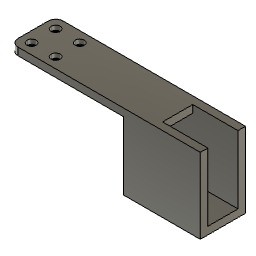
_Motor mount.45995b92-4b40-4a62-bec2-e495f78e715f (Autodesk Fusion 360 design; units mm, degrees)
Autodesk Fusion 360 part; units mm, degrees
sketch "Sketch1" plane through (0, 0, 0) normal (0, 0, 1) x (1, 0, 0)
  line L0 (0, 0) -> (51, 0)
  line L1 (51, 0) -> (51, -30)
  line L2 (51, -30) -> (0, -30)
  line L3 (0, -30) -> (0, 0)
  dimension "d1" = 51
  dimension "d2" = 30
  constraint horizontal L0
  constraint vertical L1
  constraint horizontal L2
  constraint vertical L3
  constraint coincident L0.start L3.end
  measures "d1" distance of L0.start L0.end
  measures "d2" distance of L0.start L2.end
extrude "Extrude1" add sketch "Sketch1" along normal blind 50
sketch "Sketch2" plane through (51, 0, 0) normal (1, 0, 0) x (0, 1, 0)
  line L0 (-30, 0) -> (0, 0)
  line L1 (0, 0) -> (0, 50)
  line L2 (0, 50) -> (-30, 50)
  line L3 (-30, 50) -> (-30, 0)
  line L4 (-5, 5) -> (-25, 5)
  line L5 (-25, 5) -> (-25, 45)
  line L6 (-25, 45) -> (-5, 45)
  line L7 (-5, 45) -> (-5, 5)
  dimension "d5" = 20
  dimension "d6" = 40
  constraint horizontal L4
  constraint vertical L5
  constraint horizontal L6
  constraint vertical L7
  measures "d5" distance of L4.start L4.end
  measures "d6" distance of L4.start L6.end
extrude "Extrude2" cut sketch "Sketch2" against normal blind 46 contours L4 L5 L6 L7
sketch "Sketch3" plane through (0, 0, 50) normal (0, 0, 1) x (-1, 0, 0)
  line L0 (0, 30) -> (-51, 30)
  line L1 (-51, 30) -> (-51, 0)
  line L2 (-51, 0) -> (0, 0)
  line L3 (0, 0) -> (0, 30)
  line L4 (-51, 5) -> (-21, 5)
  line L5 (-21, 5) -> (-21, 25)
  line L6 (-21, 25) -> (-51, 25)
  line L7 (-51, 25) -> (-51, 5)
  dimension "d9" = 30
  dimension "d10" = 20
  constraint horizontal L4
  constraint vertical L5
  constraint horizontal L6
  constraint vertical L7
  constraint coincident L1 L4.start
  measures "d9" distance of L4.start L4.end
  measures "d10" distance of L4.start L6.end
extrude "Extrude3" cut sketch "Sketch3" against normal blind 6 contours L1 L4 L5 L6 L7
sketch "Sketch4" plane through (0, 0, 50) normal (0, 0, 1) x (-1, 0, 0)
  line L0 (-51, 25) -> (-21, 25)
  line L1 (-21, 25) -> (-21, 5)
  line L2 (-21, 5) -> (-51, 5)
  line L3 (-51, 5) -> (-51, 0)
  line L4 (-51, 0) -> (0, 0)
  line L5 (0, 0) -> (0, 30)
  line L6 (0, 30) -> (-51, 30)
  line L7 (-51, 30) -> (-51, 25)
  line L8 (0, 0) -> (75, 0)
  line L9 (75, 0) -> (75, 30)
  line L10 (75, 30) -> (0, 30)
  line L11 (0, 30) -> (0, 0)
  dimension "d13" = 75
  dimension "d14" = 30
  constraint horizontal L8
  constraint vertical L9
  constraint horizontal L10
  constraint vertical L11
  constraint coincident L4.end L5.start
  measures "d13" distance of L4.end L8.end
  measures "d14" distance of L4.end L5.end
extrude "Extrude4" add sketch "Sketch4" against normal blind 5 contours L5 L8 L9 L10 L11
sketch "Sketch5" plane through (0, 0, 50) normal (0, 0, 1) x (-1, 0, 0)
  line L0 (-51, 25) -> (-21, 25)
  line L1 (-21, 25) -> (-21, 5)
  line L2 (-21, 5) -> (-51, 5)
  line L3 (-51, 5) -> (-51, 0)
  line L4 (-51, 0) -> (75, 0)
  line L5 (75, 0) -> (75, 30)
  line L6 (75, 30) -> (-51, 30)
  line L7 (-51, 30) -> (-51, 25)
  circle A0 centre (68, 7) radius 3
  circle A1 centre (68, 23) radius 3
  circle A2 centre (52, 7) radius 3
  circle A3 centre (52, 23) radius 3
  dimension "d17" = 6
  dimension "d18" = 6
  dimension "d19" = 6
  dimension "d20" = 6
  measures "d17" diameter of A0
  measures "d18" diameter of A1
  measures "d19" diameter of A2
  measures "d20" diameter of A3
extrude "Extrude5" cut sketch "Sketch5" against normal blind 5 contours A0 | A1 | A2 | A3
sketch "Sketch6" plane through (0, 0, 45) normal (0, 0, -1) x (1, 0, 0)
  circle A0 centre (-68, 23) radius 3
  circle A1 centre (-68, 7) radius 3
  circle A2 centre (-52, 23) radius 3
  circle A3 centre (-52, 7) radius 3
  line L0 (0, 0) -> (0, 30)
  line L1 (0, 30) -> (-75, 30)
  line L2 (-75, 30) -> (-75, 0)
  line L3 (-75, 0) -> (0, 0)
  circle A4 centre (-68, 23) radius 5
  circle A5 centre (-52, 23) radius 5
  circle A6 centre (-68, 7) radius 5
  circle A7 centre (-52, 7) radius 5
  dimension "d23" = 10
  dimension "d24" = 10
  dimension "d25" = 10
  dimension "d26" = 10
  constraint concentric A0 A4
  constraint concentric A2 A5
  constraint concentric A1 A6
  constraint concentric A3 A7
  measures "d23" diameter of A4
  measures "d24" diameter of A5
  measures "d25" diameter of A6
  measures "d26" diameter of A7
extrude "Extrude6" cut sketch "Sketch6" against normal blind 2 contours A4 | A5 | A6 | A7
fillet "Fillet1" radius 5 2 edges at (-75, -30, 47.5) (-75, 0, 47.5)
